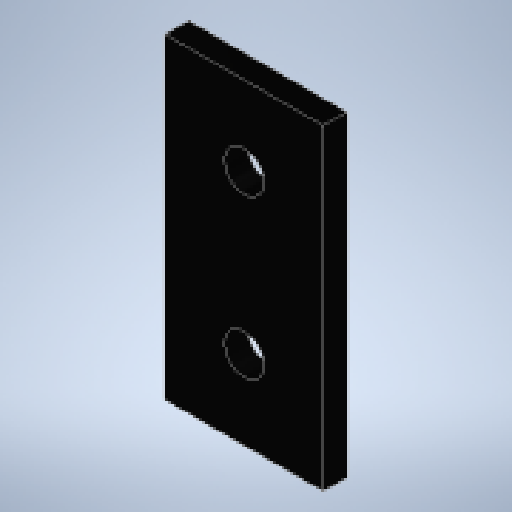
# Autodesk Inventor part: EndCap
Saved by Autodesk Inventor 2025.1 (Build 291241020, 241B)
## iProperties
Created: 2024-11-14
Part Number: EndCap
Material: Aluminum 6061
Document SubType Name: Modeling
Designer: leon-
Density: 2.7 g/cm^3
Appearance: Anodized - Black
Author: leon-
Autodesk Inventor part; units mm, degrees
ref_plane "YZ Plane" through (0, 0, 0) normal (1, 0, 0) x (0, 1, 0)
ref_plane "XZ Plane" through (0, 0, 0) normal (0, 1, 0) x (-1, 0, 0)
ref_plane "XY Plane" through (0, 0, 0) normal (0, 0, 1) x (1, 0, 0)
sketch "Sketch1" plane through (0, 0, 0) normal (0, 0, 1) x (1, 0, 0)
  line L0 (0, 0) -> (20, 0)
  line L1 (20, 0) -> (20, 40)
  line L2 (20, 40) -> (0, 40)
  line L3 (0, 40) -> (0, 0)
  circle A0 centre (10, 30) radius 2.5
  circle A1 centre (10, 10) radius 2.5
  dimension "d0" = 40
  dimension "d1" = 20
  dimension "d2" = 5
  dimension "d3" = 20
  dimension "d4" = 10
  dimension "d5" = 10
  constraints: 8 end point, 2 centre point, 2 parallel, 1 equal radius, 1 horizontal, 1 perpendicular, 1 vertical alignment
  measures "d0" distance of L0.end L1.end
  measures "d1" distance of L1.end L2.end
  measures "d2" diameter of A0
  measures "d3" distance of A1.centre A0.centre
  measures "d4" distance from line of L3 A1.centre
  measures "d5" distance from line of L0 A1.centre
extrude "Extrusion1" add sketch "Sketch1" along normal blind 3
body "Solid1"
